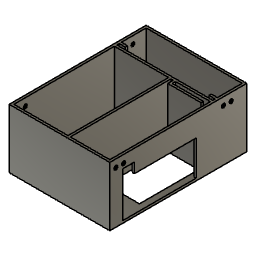
배터리 박스 테스트 (Autodesk Fusion 360 design; units mm, degrees)
Autodesk Fusion 360 part; units mm, degrees
sketch "스케치1" plane through (0, 0, 0) normal (0, 0, 1) x (1, 0, 0)
  line L0 (66.5, 88.5) -> (-66.5, 88.5)
  line L1 (-66.5, 88.5) -> (-66.5, -88.5)
  line L2 (-66.5, -88.5) -> (66.5, -88.5)
  line L3 (66.5, -88.5) -> (66.5, 88.5)
  line L4 (66.5, 88.5) -> (-66.5, -88.5) construction
  line L5 (-66.5, 88.5) -> (66.5, -88.5) construction
  line L6 (-63.5, -85.5) -> (63.5, -85.5)
  line L7 (63.5, -85.5) -> (63.5, 85.5)
  line L8 (63.5, 85.5) -> (-63.5, 85.5)
  line L9 (-63.5, 85.5) -> (-63.5, -85.5)
  line L10 (-63.5, -85.5) -> (63.5, 85.5) construction
  line L11 (63.5, -85.5) -> (-63.5, 85.5) construction
  line L12 (-63.5, 0) -> (6.5, 0)
  line L13 (6.5, 0) -> (9.5, 0)
  line L14 (9.5, 0) -> (55.5, 0)
  line L15 (6.5, 0) -> (6.5, -85.5)
  line L16 (6.5, -85.5) -> (-63.5, -85.5)
  line L17 (-63.5, -85.5) -> (-63.5, 44.5)
  line L18 (-63.5, 44.5) -> (6.5, 44.5)
  line L19 (6.5, 44.5) -> (6.5, -85.5)
  line L20 (-63.5, 44.5) -> (6.5, 44.5)
  line L21 (6.5, 44.5) -> (6.5, 47.5)
  line L22 (6.5, 47.5) -> (-63.5, 47.5)
  line L23 (-63.5, 47.5) -> (-63.5, 44.5)
  line L24 (6.5, 47.5) -> (9.5, 47.5)
  line L25 (9.5, 47.5) -> (9.5, -85.5)
  line L26 (9.5, -85.5) -> (6.5, -85.5)
  line L27 (6.5, -85.5) -> (6.5, 47.5)
  line L28 (55.5, -85.5) -> (9.5, -85.5)
  line L29 (9.5, -85.5) -> (9.5, 26.5)
  line L30 (9.5, 26.5) -> (55.5, 26.5)
  line L31 (55.5, 26.5) -> (55.5, -85.5)
  line L32 (55.5, 26.5) -> (9.5, 26.5)
  line L33 (9.5, 26.5) -> (9.5, -33.5)
  line L34 (9.5, -33.5) -> (55.5, -33.5)
  line L35 (55.5, -33.5) -> (55.5, 26.5)
  line L36 (55.5, 26.5) -> (12.5, 26.5)
  line L37 (-63.5, 47.5) -> (-63.5, 50.5)
  line L38 (-63.5, 50.5) -> (-55.5, 50.5)
  line L39 (-55.5, 50.5) -> (-55.5, 53.5)
  line L40 (-55.5, 53.5) -> (-63.5, 53.5)
  line L41 (-63.5, 53.5) -> (-63.5, 50.5)
  line L42 (63.5, 47.5) -> (63.5, 50.5)
  line L43 (63.5, 50.5) -> (52.5, 50.5)
  line L44 (52.5, 50.5) -> (52.5, 53.5)
  line L45 (52.5, 53.5) -> (63.5, 53.5)
  line L46 (63.5, 53.5) -> (63.5, 50.5)
  line L47 (63.5, 47.5) -> (52.5, 47.5)
  line L48 (52.5, 47.5) -> (52.5, 44.5)
  line L49 (52.5, 44.5) -> (63.5, 44.5)
  line L50 (63.5, 44.5) -> (63.5, 47.5)
  line L51 (63.5, 85.5) -> (60.5, 85.5)
  line L52 (60.5, 85.5) -> (60.5, -85.5)
  line L53 (60.5, -85.5) -> (63.5, -85.5)
  line L54 (63.5, -85.5) -> (63.5, 85.5)
  line L55 (63.5, -85.5) -> (63.5, -88.5)
  line L56 (63.5, 85.5) -> (63.5, 88.5)
  line L57 (52.5, 47.5) -> (9.5, 47.5)
  line L58 (9.5, 47.5) -> (9.5, 44.5)
  line L59 (9.5, 44.5) -> (52.5, 44.5)
  line L60 (52.5, 44.5) -> (52.5, 47.5)
  line L61 (9.5, 44.5) -> (12.5, 44.5)
  line L62 (12.5, 44.5) -> (15.5, 44.5)
  line L63 (15.5, 44.5) -> (15.5, 40.3)
  line L64 (15.5, 40.3) -> (12.5, 40.3)
  line L65 (12.5, 40.3) -> (12.5, 44.5)
  line L66 (12.5, 40.3) -> (55.5, 40.3)
  line L67 (55.5, 40.3) -> (55.5, 37.3)
  line L68 (55.5, 37.3) -> (12.5, 37.3)
  line L69 (12.5, 37.3) -> (12.5, 40.3)
  dimension "d1" = 133
  dimension "d2" = 177
  dimension "d3" = 127
  dimension "d4" = 171
  dimension "d22" = 70
  dimension "d23" = 3
  dimension "d24" = 46
  dimension "d25" = 130
  dimension "d26" = 3
  dimension "d27" = 3
  dimension "d28" = 46
  dimension "d29" = 112
  dimension "d30" = 46
  dimension "d31" = 60
  dimension "d44" = 3
  dimension "d45" = 8
  dimension "d46" = 3
  dimension "d47" = 3
  dimension "d48" = 11
  dimension "d49" = 3
  dimension "d50" = 11
  dimension "d51" = 3
  dimension "d54" = 3
  dimension "d111" = 3
  dimension "d112" = 3
  dimension "d113" = 3
  dimension "d114" = 4.2
  dimension "d115" = 3
  constraint horizontal L0
  constraint perpendicular L0 L1
  constraint parallel L0 L2
  constraint parallel L1 L3
  constraint coincident L4 origin
  constraint coincident L5 origin
  constraint horizontal L6
  constraint perpendicular L6 L7
  constraint parallel L6 L8
  constraint parallel L7 L9
  constraint coincident L10 origin
  constraint coincident L11 origin
  constraint midpoint L9 L12.start
  constraint perpendicular L9 L12
  constraint parallel L12 L13
  constraint parallel L13 L14
  constraint coincident L6 L15.end
  constraint perpendicular L6 L15
  constraint horizontal L16
  constraint vertical L17
  constraint horizontal L18
  constraint vertical L19
  constraint horizontal L20
  constraint vertical L21
  constraint horizontal L22
  constraint vertical L23
  constraint horizontal L24
  constraint vertical L25
  constraint horizontal L26
  constraint vertical L27
  constraint coincident L6 L25.end
  constraint horizontal L28
  constraint vertical L29
  constraint horizontal L30
  constraint vertical L31
  constraint coincident L6 L28.start
  constraint horizontal L32
  constraint vertical L33
  constraint horizontal L34
  constraint vertical L35
  constraint horizontal L36
  constraint perpendicular L22 L37
  constraint horizontal L38
  constraint vertical L39
  constraint horizontal L40
  constraint vertical L41
  constraint coincident L7 L42.start
  constraint parallel L7 L42
  constraint horizontal L43
  constraint vertical L44
  constraint horizontal L45
  constraint vertical L46
  constraint horizontal L47
  constraint vertical L48
  constraint horizontal L49
  constraint vertical L50
  constraint horizontal L51
  constraint vertical L52
  constraint horizontal L53
  constraint vertical L54
  constraint coincident L6 L52.end
  constraint coincident L2 L55.end
  constraint perpendicular L2 L55
  constraint coincident L0 L56.end
  constraint perpendicular L0 L56
  constraint horizontal L57
  constraint vertical L58
  constraint horizontal L59
  constraint vertical L60
  constraint perpendicular L58 L61
  constraint horizontal L62
  constraint vertical L63
  constraint horizontal L64
  constraint vertical L65
  constraint horizontal L66
  constraint vertical L67
  constraint horizontal L68
  constraint vertical L69
  measures "d1" distance of L1.end L2.end
  measures "d2" distance of L0.end L1.end
  measures "d3" distance of L7.end L8.end
  measures "d4" distance of L6.end L7.end
  measures "d22" distance of L12.start L12.end
  measures "d23" distance of L12.end L13.end
  measures "d24" distance of L13.end L14.end
  measures "d25" distance of L15.end L18.end
  measures "d26" distance of L17.end L22.end
  measures "d27" distance of L21.end L24.end
  measures "d28" distance of L28.start L25.end
  measures "d29" distance of L28.start L30.end
  measures "d30" distance of L30.end L29.end
  measures "d31" distance of L30.end L34.end
  measures "d44" distance of L22.end L37.end
  measures "d45" distance of L37.end L38.end
  measures "d46" distance of L37.end L40.end
  measures "d47" distance of L42.start L42.end
  measures "d48" distance of L42.end L43.end
  measures "d49" distance of L42.end L45.end
  measures "d50" distance of L42.start L47.end
  measures "d51" distance of L42.start L49.end
  measures "d54" distance of L7.end L51.end
  measures "d111" distance of L47.end L48.end
  measures "d112" distance of L58.end L61.end
  measures "d113" distance of L61.end L62.end
  measures "d114" distance of L61.end L64.end
  measures "d115" distance of L64.end L68.end
extrude "돌출4" add sketch "스케치1" along normal blind 76.5 contours L0 L1 L2 L6 L8 L9 L16 L17 L23 L26 L28 L37 L41 L51 L53 L55 L56
extrude "돌출5" add sketch "스케치1" along normal blind 3 contours L7 L8 L45 L51 L52 L54 | L7 L43 L45 L46 L52 L54 | L8 L9 L22 L24 L37 L38 L39 L40 L43 L44 L45 L47 L52 L57 | L6 L7 L49 L52 L53 L54 | L7 L42 L43 L47 L52 L54 | L43 L44 L45 L52 | L6 L25 L30 L31 L32 L35 L36 L49 L52 L59 L61 L63 L65 L66 L67 L68 L69 | L7 L47 L49 L50 L52 L54 | L9 L38 L39 L40 L41 | L6 L25 L28 L29 L31 L34 | L47 L48 L49 L52 L60 | L14 L25 L29 L31 L33 L34 L35 | L25 L48 L57 L58 L59 L60 L61 L62 | L6 L9 L12 L15 L16 L17 L19 L27 | L59 L62 L63 L64 L65 L66 | L9 L12 L17 L18 L19 L20 L27 | L64 L66 L67 L68 L69
extrude "돌출6" add sketch "스케치1" along normal blind 76.5 contours L7 L43 L45 L46 L52 L54 | L43 L44 L45 L52 | L7 L47 L49 L50 L52 L54 | L9 L38 L39 L40 L41 | L47 L48 L49 L52 L60 | L6 L13 L15 L19 L25 L26 L27 L29 L33 | L25 L48 L57 L58 L59 L60 L61 L62 | L9 L18 L20 L21 L22 L23 L27 | L59 L62 L63 L64 L65 L66 | L13 L19 L21 L24 L25 L27 L29 L33 L58 | L64 L66 L67 L68 L69
extrude "돌출7" cut 1 faces at (24.8333, 0, 1) along direction (0, -1, 0) blind 53
extrude "돌출8" add sketch "스케치1" along normal blind 76.5 contours L7 L8 L45 L51 L52 L54 | L7 L43 L45 L46 L52 L54 | L6 L7 L49 L52 L53 L54 | L7 L42 L43 L47 L52 L54 | L7 L47 L49 L50 L52 L54
sketch "스케치3" plane through (-66.5, 0, 0) normal (-1, 0, 0) x (0, -1, 0)
  line L0 (-88.5, 0) -> (88.5, 0)
  line L1 (88.5, 0) -> (88.5, 76.5)
  line L2 (88.5, 76.5) -> (-88.5, 76.5)
  line L3 (-88.5, 76.5) -> (-88.5, 0)
  line L4 (88.5, 76.5) -> (65.5, 76.5)
  line L5 (65.5, 76.5) -> (65.5, 61.5)
  line L6 (65.5, 61.5) -> (88.5, 61.5)
  line L7 (88.5, 61.5) -> (88.5, 76.5)
  line L8 (65.5, 76.5) -> (88.5, 76.5)
  line L9 (88.5, 76.5) -> (88.5, 71.5)
  line L10 (88.5, 71.5) -> (65.5, 71.5)
  line L11 (65.5, 71.5) -> (65.5, 76.5)
  line L12 (65.5, 61.5) -> (70.5, 61.5)
  line L13 (70.5, 61.5) -> (70.5, 66.5)
  line L14 (70.5, 66.5) -> (65.5, 66.5)
  line L15 (65.5, 66.5) -> (65.5, 61.5)
  circle A0 centre (70.5, 66.5) radius 2.65
  line L16 (88.5, 61.5) -> (80.5, 61.5)
  line L17 (80.5, 61.5) -> (80.5, 66.5)
  line L18 (80.5, 66.5) -> (88.5, 66.5)
  line L19 (88.5, 66.5) -> (88.5, 61.5)
  circle A1 centre (80.5, 66.5) radius 2.65
  line L20 (-88.5, 76.5) -> (-53.5, 76.5)
  line L21 (-53.5, 76.5) -> (-53.5, 61.5)
  line L22 (-53.5, 61.5) -> (-88.5, 61.5)
  line L23 (-88.5, 61.5) -> (-88.5, 76.5)
  line L24 (-53.5, 76.5) -> (-73.5, 76.5)
  line L25 (-73.5, 76.5) -> (-73.5, 61.5)
  line L26 (-73.5, 61.5) -> (-53.5, 61.5)
  line L27 (-53.5, 61.5) -> (-53.5, 76.5)
  line L28 (-73.5, 61.5) -> (-68.5, 61.5)
  line L29 (-68.5, 61.5) -> (-68.5, 66.5)
  line L30 (-68.5, 66.5) -> (-73.5, 66.5)
  line L31 (-73.5, 66.5) -> (-73.5, 61.5)
  line L32 (-53.5, 61.5) -> (-58.5, 61.5)
  line L33 (-58.5, 61.5) -> (-58.5, 66.5)
  line L34 (-58.5, 66.5) -> (-53.5, 66.5)
  line L35 (-53.5, 66.5) -> (-53.5, 61.5)
  circle A2 centre (-68.5, 66.5) radius 2.65
  circle A3 centre (-58.5, 66.5) radius 2.65
  dimension "d57" = 23
  dimension "d58" = 15
  dimension "d59" = 5
  dimension "d60" = 5
  dimension "d61" = 5
  dimension "d62" = 5.3
  dimension "d63" = 8
  dimension "d64" = 5
  dimension "d65" = 5.3
  dimension "d66" = 35
  dimension "d67" = 15
  dimension "d68" = 20
  dimension "d69" = 5
  dimension "d70" = 5
  dimension "d71" = 5
  dimension "d72" = 5
  dimension "d73" = 5.3
  dimension "d74" = 5.3
  constraint horizontal L4
  constraint vertical L5
  constraint horizontal L6
  constraint vertical L7
  constraint coincident L1.end L2.start
  constraint horizontal L8
  constraint vertical L9
  constraint horizontal L10
  constraint vertical L11
  constraint horizontal L12
  constraint vertical L13
  constraint horizontal L14
  constraint vertical L15
  constraint coincident L13.end L14.start
  constraint horizontal L16
  constraint vertical L17
  constraint horizontal L18
  constraint vertical L19
  constraint coincident L17.end L18.start
  constraint horizontal L20
  constraint vertical L21
  constraint horizontal L22
  constraint vertical L23
  constraint coincident L2.end L3.start
  constraint horizontal L24
  constraint vertical L25
  constraint horizontal L26
  constraint vertical L27
  constraint horizontal L28
  constraint vertical L29
  constraint horizontal L30
  constraint vertical L31
  constraint horizontal L32
  constraint vertical L33
  constraint horizontal L34
  constraint vertical L35
  constraint coincident L29.end L30.start
  constraint coincident L33.end L34.start
  measures "d57" distance of L1.end L4.end
  measures "d58" distance of L1.end L6.end
  measures "d59" distance of L4.end L10.end
  measures "d60" distance of L5.end L12.end
  measures "d61" distance of L5.end L14.end
  measures "d62" diameter of A0
  measures "d63" distance of L6.end L16.end
  measures "d64" distance of L6.end L18.end
  measures "d65" diameter of A1
  measures "d66" distance of L2.end L20.end
  measures "d67" distance of L2.end L22.end
  measures "d68" distance of L20.end L24.end
  measures "d69" distance of L25.end L28.end
  measures "d70" distance of L25.end L30.end
  measures "d71" distance of L21.end L32.end
  measures "d72" distance of L21.end L34.end
  measures "d73" diameter of A2
  measures "d74" diameter of A3
extrude "돌출9" cut sketch "스케치3" against normal blind 3 contours L17 L18 A1 | L17 L18 A1 | L29 L30 A2 | L29 L30 A2 | L13 L14 A0 | L13 L14 A0 | L33 L34 A3 | L33 L34 A3
sketch "스케치4" plane through (63.5, 0, 0) normal (1, 0, 0) x (0, 1, 0)
  line L0 (88.5, 76.5) -> (-88.5, 76.5)
  line L1 (-88.5, 76.5) -> (-88.5, 0)
  line L2 (-88.5, 0) -> (88.5, 0)
  line L3 (88.5, 0) -> (88.5, 76.5)
  line L4 (-88.5, 76.5) -> (-65.5, 76.5)
  line L5 (-65.5, 76.5) -> (-65.5, 61.5)
  line L6 (-65.5, 61.5) -> (-88.5, 61.5)
  line L7 (-88.5, 61.5) -> (-88.5, 76.5)
  line L8 (-65.5, 61.5) -> (-70.5, 61.5)
  line L9 (-70.5, 61.5) -> (-70.5, 66.5)
  line L10 (-70.5, 66.5) -> (-65.5, 66.5)
  line L11 (-65.5, 66.5) -> (-65.5, 61.5)
  line L12 (-88.5, 61.5) -> (-80.5, 61.5)
  line L13 (-80.5, 61.5) -> (-80.5, 66.5)
  line L14 (-80.5, 66.5) -> (-88.5, 66.5)
  line L15 (-88.5, 66.5) -> (-88.5, 61.5)
  circle A0 centre (-80.5, 66.5) radius 2.65
  circle A1 centre (-70.5, 66.5) radius 2.65
  line L16 (88.5, 76.5) -> (53.5, 76.5)
  line L17 (53.5, 76.5) -> (53.5, 61.5)
  line L18 (53.5, 61.5) -> (88.5, 61.5)
  line L19 (88.5, 61.5) -> (88.5, 76.5)
  line L20 (53.5, 61.5) -> (58.5, 61.5)
  line L21 (58.5, 61.5) -> (58.5, 66.5)
  line L22 (58.5, 66.5) -> (53.5, 66.5)
  line L23 (53.5, 66.5) -> (53.5, 61.5)
  line L24 (53.5, 76.5) -> (73.5, 76.5)
  line L25 (73.5, 76.5) -> (73.5, 61.5)
  line L26 (73.5, 61.5) -> (53.5, 61.5)
  line L27 (53.5, 61.5) -> (53.5, 76.5)
  line L28 (73.5, 61.5) -> (68.5, 61.5)
  line L29 (68.5, 61.5) -> (68.5, 66.5)
  line L30 (68.5, 66.5) -> (73.5, 66.5)
  line L31 (73.5, 66.5) -> (73.5, 61.5)
  circle A2 centre (68.5, 66.5) radius 2.65
  circle A3 centre (58.5, 66.5) radius 2.65
  dimension "d77" = 23
  dimension "d78" = 15
  dimension "d79" = 5
  dimension "d80" = 8
  dimension "d81" = 5
  dimension "d82" = 5.3
  dimension "d83" = 5.3
  dimension "d84" = 35
  dimension "d85" = 15
  dimension "d86" = 5
  dimension "d87" = 5
  dimension "d88" = 20
  dimension "d89" = 15
  dimension "d90" = 5
  dimension "d91" = 5
  dimension "d92" = 5.3
  dimension "d93" = 5.3
  constraint horizontal L4
  constraint vertical L5
  constraint horizontal L6
  constraint vertical L7
  constraint coincident L0.end L1.start
  constraint horizontal L8
  constraint vertical L9
  constraint horizontal L10
  constraint vertical L11
  constraint horizontal L12
  constraint vertical L13
  constraint horizontal L14
  constraint vertical L15
  constraint coincident L13.end L14.start
  constraint coincident L9.end L10.start
  constraint horizontal L16
  constraint vertical L17
  constraint horizontal L18
  constraint vertical L19
  constraint coincident L0.start L3.end
  constraint horizontal L20
  constraint vertical L21
  constraint horizontal L22
  constraint vertical L23
  constraint horizontal L24
  constraint vertical L25
  constraint horizontal L26
  constraint vertical L27
  constraint horizontal L28
  constraint vertical L29
  constraint horizontal L30
  constraint vertical L31
  constraint coincident L29.end L30.start
  constraint coincident L21.end L22.start
  measures "d77" distance of L0.end L4.end
  measures "d78" distance of L0.end L6.end
  measures "d79" distance of L5.end L8.end
  measures "d80" distance of L6.end L12.end
  measures "d81" distance of L6.end L14.end
  measures "d82" diameter of A0
  measures "d83" diameter of A1
  measures "d84" distance of L0.start L16.end
  measures "d85" distance of L0.start L18.end
  measures "d86" distance of L17.end L20.end
  measures "d87" distance of L17.end L22.end
  measures "d88" distance of L16.end L24.end
  measures "d89" distance of L16.end L17.end
  measures "d90" distance of L25.end L28.end
  measures "d91" distance of L25.end L30.end
  measures "d92" diameter of A2
  measures "d93" diameter of A3
extrude "돌출10" cut sketch "스케치4" against normal blind 3 contours L29 L30 A2 | L29 L30 A2 | L21 L22 A3 | L21 L22 A3 | L9 L10 A1 | L9 L10 A1 | L13 L14 A0 | L13 L14 A0
thread "나사산2" "ISO Metric profile 5.0 M5x0.8 6H" major diameter 5.12 minor diameter 4.234 pitch 0.8 angle 60 modelled right hand crest width 0.2219 on face at (62.5, 66.9531, 64.3484) crest through (63.3, 70.617, 66.5) on face at (-64.5, 56.1727, 67.7674) crest through (-66.3, 56.383, 66.5) on face at (-64.5, 70.7612, 65.1182) crest through (-66.3, 66.383, 66.5) on face at (-64.5, -78.2388, 65.1182) crest through (-66.3, -82.617, 66.5) on face at (-64.5, -68.2388, 65.1182) crest through (-66.3, -72.617, 66.5) on face at (61.5, -82.7612, 65.1182) crest through (63.3, -78.383, 66.5) on face at (61.5, -72.53, 64.7966) crest through (63.3, -68.383, 66.5) on face at (62.5, 61.1368, 66.7639) crest through (63.3, 60.617, 66.5)
sketch "스케치6" plane through (60.5, 0, 0) normal (-1, 0, 0) x (0, -1, 0)
  spline S0 degree 3 poles (71.8629, 64.8801) (71.6688, 64.6789) (71.4366, 64.5184) (70.9143, 64.2889) (70.6276, 64.226) (70.0351, 64.2114) (69.7349, 64.2639) (69.1603, 64.4832) (68.893, 64.6517) (68.5234, 64.9987) (68.3984, 65.1477) (68.1831, 65.4748) (68.0943, 65.6523) (68.027, 65.8383) knots 0 0 0 0 0.083865 0.083865 0.170995 0.170995 0.261388 0.261388 0.355043 0.355043 0.412991 0.412991 0.47212 0.47212 0.47212 0.47212
  arc A0 (68.027, 67.1617) -> (68.027, 65.8383) centre (70.5, 66.5) ccw
  spline S1 degree 3 poles (68.027, 67.1617) (68.1383, 67.469) (68.3075, 67.752) (68.7391, 68.2276) (68.9941, 68.4184) (69.5538, 68.6849) (69.8513, 68.7618) (70.4481, 68.7945) (70.7413, 68.7542) (71.1794, 68.6019) (71.3335, 68.5273) (71.6176, 68.3456) (71.7472, 68.2399) (71.8629, 68.1199) knots 0 0 0 0 0.098035 0.098035 0.192799 0.192799 0.284291 0.284291 0.372508 0.372508 0.423853 0.423853 0.474023 0.474023 0.474023 0.474023
  arc A1 (71.8629, 64.8801) -> (71.8629, 68.1199) centre (70.5, 66.5) ccw
  spline S2 degree 3 poles (81.8629, 64.8801) (81.6688, 64.6789) (81.4366, 64.5184) (80.9143, 64.2889) (80.6276, 64.226) (80.0351, 64.2114) (79.7349, 64.2639) (79.1603, 64.4832) (78.893, 64.6517) (78.5234, 64.9987) (78.3984, 65.1477) (78.1831, 65.4748) (78.0943, 65.6523) (78.027, 65.8383) knots 0 0 0 0 0.083865 0.083865 0.170995 0.170995 0.261388 0.261388 0.355043 0.355043 0.412991 0.412991 0.47212 0.47212 0.47212 0.47212
  arc A2 (78.027, 67.1617) -> (78.027, 65.8383) centre (80.5, 66.5) ccw
  spline S3 degree 3 poles (78.027, 67.1617) (78.1383, 67.469) (78.3075, 67.752) (78.7391, 68.2276) (78.9941, 68.4184) (79.5538, 68.6849) (79.8513, 68.7618) (80.4481, 68.7945) (80.7413, 68.7542) (81.1794, 68.6019) (81.3335, 68.5273) (81.6176, 68.3456) (81.7472, 68.2399) (81.8629, 68.1199) knots 0 0 0 0 0.098035 0.098035 0.192799 0.192799 0.284291 0.284291 0.372508 0.372508 0.423853 0.423853 0.474023 0.474023 0.474023 0.474023
  arc A3 (81.8629, 64.8801) -> (81.8629, 68.1199) centre (80.5, 66.5) ccw
  line L0 (-44.5, 3) -> (85.5, 3)
  line L1 (85.5, 3) -> (85.5, 76.5)
  line L2 (85.5, 76.5) -> (-44.5, 76.5)
  line L3 (-44.5, 76.5) -> (-44.5, 3)
  line L4 (85.5, 3) -> (82.5, 3)
  line L5 (82.5, 3) -> (67.5, 3)
  line L6 (67.5, 3) -> (67.5, 61)
  line L7 (67.5, 61) -> (82.5, 61)
  line L8 (82.5, 61) -> (82.5, 3)
  line L9 (67.5, 3) -> (-12.5, 3)
  line L10 (-12.5, 3) -> (-12.5, 48)
  line L11 (-12.5, 48) -> (67.5, 48)
  line L12 (67.5, 48) -> (67.5, 3)
  dimension "d100" = 3
  dimension "d101" = 15
  dimension "d102" = 58
  dimension "d103" = 80
  dimension "d104" = 45
  constraint coincident L0.end L1.start
  constraint perpendicular L1 L4
  constraint horizontal L5
  constraint vertical L6
  constraint horizontal L7
  constraint vertical L8
  constraint horizontal L9
  constraint vertical L10
  constraint horizontal L11
  constraint vertical L12
  measures "d100" distance of L0.end L4.end
  measures "d101" distance of L4.end L5.end
  measures "d102" distance of L4.end L7.end
  measures "d103" distance of L5.end L9.end
  measures "d104" distance of L5.end L11.end
extrude "돌출12" cut sketch "스케치6" against normal blind 15 contours L0 L6 L9 L10 L11 L12 | L0 L5 L6 L7 L8 L12
extrude "돌출15" cut 1 faces at (24.8333, 26.5, 1) along direction (0, 1, 0) blind 10.8
extrude "돌출16" add 1 faces at (24.8333, -53, 1) along direction (0, 1, 0) blind 10.8
extrude "돌출17" cut 1 faces at (62.5, 12.5, 18) along direction (0, 1, 0) blind 10.8
extrude "돌출18" cut 1 faces at (61.5, -67.5, 52.3333) along direction (0, 1, 0) blind 10.8
extrude "돌출19" add 1 faces at (61.5, -82.5, 41.6667) along direction (0, 1, 0) blind 10.8
